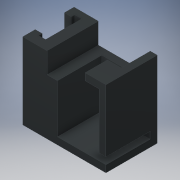
# Autodesk Inventor part: Holder
Saved by Autodesk Inventor 2017 (Build 210142000, 142)
## iProperties
Created: 2017-05-30
Part Number: Holder
Material: Iron, Cast
Document SubType Name: Modeling
Designer: sensor
Density: 7.15 g/cm^3
Appearance: Iron Gray
Author: sensor
Autodesk Inventor part; units mm, degrees
ref_plane "YZ Plane" through (0, 0, 0) normal (1, 0, 0) x (0, 1, 0)
ref_plane "XZ Plane" through (0, 0, 0) normal (0, 1, 0) x (-1, 0, 0)
ref_plane "XY Plane" through (0, 0, 0) normal (0, 0, 1) x (1, 0, 0)
sketch "Sketch3" plane through (0, 0, 0) normal (0, 0, 1) x (1, 0, 0)
  line L0 (0, 0) -> (0, 55)
  line L1 (0, 55) -> (17.5, 55)
  line L2 (17.5, 55) -> (17.5, 40)
  line L3 (17.5, 40) -> (45, 40)
  line L4 (45, 40) -> (45, 55)
  line L5 (10.4377, 0) -> (0, 0)
  line L6 (45, 55) -> (60, 55)
  line L7 (60, 55) -> (60, 0)
  line L8 (60, 0) -> (0, 0)
  dimension "d7" = 55
  dimension "d8" = 17.5
  dimension "d12" = 15
  dimension "d13" = 27.5
  dimension "d14" = 15
  dimension "d15" = 55
  dimension "d16" = 60
  constraints: 18 end point, 4 perpendicular, 2 vertical, 1 collinear, 1 horizontal, 1 point on line
  measures "d7" distance of L0.start L0.end
  measures "d8" distance of L0.end L1.end
  measures "d12" distance of L1.end L2.end
  measures "d13" distance of L2.end L3.end
  measures "d14" distance of L4.end L6.end
  measures "d15" distance of L6.end L7.end
  measures "d16" distance of L7.end L0.start
extrude "Extrusion2" add sketch "Sketch3" along normal blind 5
sketch "Sketch4" plane through (0, 55, 0) normal (0, 1, 0) x (1, 0, 0)
  line L0 (17.5, -5) -> (0, -5) projected
  line L1 (0, -37) -> (17.5, -37)
  line L2 (17.5, -37) -> (17.5, -5)
  line L3 (17.5, -5) -> (0, -5)
  line L4 (0, -5) -> (0, -37)
  point P0 (0, 0)
  dimension "d20" = 32
  dimension "d21" = 17.5
  constraints: 8 end point, 2 parallel, 1 horizontal, 1 perpendicular
  measures "d20" distance of L3.end L1.start
  measures "d21" distance of L1.start L1.end
extrude "Extrusion3" add sketch "Sketch4" against normal blind 55
sketch "Sketch5" plane through (45, 55, 0) normal (0, 1, 0) x (1, 0, 0)
  line L0 (15, 0) -> (15, -5) projected
  line L1 (-0.039, -37) -> (15, -37)
  line L2 (15, -37) -> (15, -5)
  line L3 (15, -5) -> (-0.039, -5)
  line L4 (-0.039, -5) -> (-0.039, -37)
  point P0 (-45, 0)
  dimension "d24" = 32
  constraints: 8 end point, 2 parallel, 1 horizontal, 1 perpendicular
  measures "d24" distance of L3.end L1.start
extrude "Extrusion4" add sketch "Sketch5" against normal blind 5
sketch "Sketch7" plane through (17.5, 40, 0) normal (0, 1, 0) x (1, 0, 0)
  line L0 (0, -5) -> (0, -37) projected
  line L1 (27.5, -5) -> (0, -5) projected
  line L2 (0, -37) -> (7.5, -37)
  line L3 (7.5, -37) -> (7.5, -5)
  line L4 (7.5, -5) -> (0, -5)
  line L5 (0, -5) -> (0, -37)
  point P0 (-17.5, 0)
  dimension "d27" = 7.5
  constraints: 8 end point, 2 parallel, 1 horizontal, 1 perpendicular, 1 point on line
  measures "d27" distance of L0.end L2.end
extrude "Extrusion5" add sketch "Sketch7" against normal blind 40
sketch "Sketch8" plane through (0, 0, 5) normal (0, 0, 1) x (1, 0, 0)
  line L0 (25, 0) -> (60, 0) projected
  line L1 (60, 0) -> (60, 50) projected
  line L2 (25, 0) -> (60, 0)
  line L3 (60, 0) -> (60, 5)
  line L4 (60, 5) -> (25, 5)
  line L5 (25, 5) -> (25, 0)
  point P0 (0, 0)
  dimension "d30" = 5
  constraints: 8 end point, 2 parallel, 1 horizontal, 1 perpendicular, 1 point on line
  measures "d30" distance of L4.end L0.start
extrude "Extrusion6" add sketch "Sketch8" along normal blind 32
sketch "Sketch9" plane through (0, 0, 5) normal (0, 0, 1) x (1, 0, 0)
  line L0 (60, 50) -> (45, 50) projected
  line L1 (60, 50) -> (55, 50)
  line L2 (55, 50) -> (55, 0)
  line L3 (55, 0) -> (60, 0)
  line L4 (60, 0) -> (60, 50)
  point P0 (0, 0)
  dimension "d31" = 32
  dimension "d33" = 50
  dimension "d34" = 5
  constraints: 8 end point, 2 parallel, 1 horizontal, 1 perpendicular
  measures "d33" distance of L1.end L2.end
  measures "d34" distance of L2.end L3.end
extrude "Extrusion7" add sketch "Sketch9" along normal blind 32
sketch "Sketch10" plane through (0, 55, 0) normal (0, 1, 0) x (1, 0, 0)
  line L0 (10, -30.5) -> (5, -30.5)
  line L1 (5, -30.5) -> (5, -4.5)
  line L2 (5, -4.5) -> (10, -4.5)
  line L3 (10, -4.5) -> (10, -30.5)
  line L4 (17.5, 0) -> (17.5, -37) projected
  line L5 (0, 0) -> (17.5, 0) projected
  line L6 (0, 0) -> (0, -37) projected
  dimension "d45" = 5
  dimension "d46" = 26
  dimension "d47" = 7.5
  dimension "d48" = 4.5
  constraints: 8 end point, 2 parallel, 1 horizontal, 1 perpendicular
  measures "d45" distance of L0.start L0.end
  measures "d46" distance of L0.end L1.end
  measures "d47" distance between parallel lines of L4 L3
  measures "d48" distance between parallel lines of L5 L2
extrude "Extrusion8" cut sketch "Sketch10" against normal blind 60
sketch "Sketch11" plane through (0, 55, 0) normal (0, 1, 0) x (1, 0, 0)
  line L0 (5, -4.5) -> (5, -30.5) projected
  line L1 (0, 0) -> (0, -37) projected
  line L2 (5, -28) -> (0, -28)
  line L3 (0, -28) -> (0, -7)
  line L4 (0, -7) -> (5, -7)
  line L5 (5, -7) -> (5, -28)
  line L6 (0, -37) -> (17.5, -37) projected
  point P0 (5, -35)
  dimension "d52" = 21
  dimension "d53" = 9
  constraints: 8 end point, 2 parallel, 2 point on line, 1 horizontal, 1 perpendicular
  measures "d52" distance between parallel lines of L4 L2
  measures "d53" distance between parallel lines of L2 L6
extrude "Extrusion9" cut sketch "Sketch11" against normal blind 60
sketch "Sketch12" plane through (0, 0, 0) normal (0, -1, 0) x (1, 0, 0)
  circle A0 centre (17.5, 10.5) radius 2.5
  circle A1 centre (17.5, 23) radius 2.5
  line L0 (10, 30.5) -> (10, 4.5) projected
  line L1 (0, 37) -> (60, 37) projected
  line L2 (60, 0) -> (0, 0) projected
  point P0 (10, 35)
  point P1 (25, 35)
  dimension "d56" = 5
  dimension "d57" = 5
  dimension "d58" = 7.5
  dimension "d59" = 7.5
  dimension "d78" = 14
  dimension "d79" = 12.5
  constraints: 2 centre point, 1 other
  measures "d56" diameter of A1
  measures "d57" diameter of A0
  measures "d58" distance from line of L0 A0.centre
  measures "d59" distance from line of L0 A1.centre
  measures "d79" distance of A0.centre A1.centre
hole "Hole1" at (17.5, 0, 10.5) at (17.5, 0, 23) direction (0, 1, 0) diameter 5.86 depth 5 tip angle 118
sketch "Sketch14" plane through (0, 55, 37) normal (0, 0, 1) x (1, 0, 0)
  line L0 (55, -5) -> (55, -50) projected
  line L1 (60, 0) -> (60, -55) projected
  line L2 (55, -50) -> (60, -50)
  line L3 (60, -50) -> (60, -45)
  line L4 (60, -45) -> (55, -45)
  line L5 (55, -45) -> (55, -50)
  point P0 (0, -55)
  dimension "d69" = 5
  constraints: 8 end point, 2 parallel, 1 horizontal, 1 perpendicular, 1 point on line
  measures "d69" distance between parallel lines of L2 L4
extrude "Extrusion10" cut sketch "Sketch14" along normal mid plane 64
sketch "Sketch20" plane through (45, 55, 0) normal (0, 1, 0) x (1, 0, 0)
  line L0 (-0.039, -37) -> (-0.039, -5) projected
  line L1 (0, 0) -> (15, 0) projected
  line L2 (-0.039, -21) -> (10, -21)
  line L3 (10, -21) -> (10, 0)
  line L4 (10, 0) -> (-0.039, 0)
  line L5 (-0.039, 0) -> (-0.039, -21)
  line L6 (15, 0) -> (15, -37) projected
  point P0 (-45, 0)
  dimension "d77" = 5
  constraints: 8 end point, 2 parallel, 1 horizontal, 1 midpoint, 1 perpendicular, 1 point on line
  measures "d77" distance between parallel lines of L6 L3
extrude "Extrusion12" cut sketch "Sketch20" against normal blind 15
body "Solid2"
